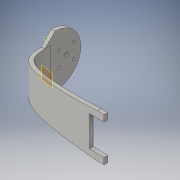
# Autodesk Inventor part: backplaterev2.0
Saved by Autodesk Inventor 2016 (Build 200138000, 138)
## iProperties
Created: 2017-03-21
Part Number: backplaterev2.0
Material: Generic
Document SubType Name: Modeling
Designer: Jorian Bruslind
Density: 1 g/cm^3
Appearance: Default
Author: Jorian Bruslind
Autodesk Inventor part; units mm, degrees
ref_plane "YZ Plane" through (0, 0, 0) normal (1, 0, 0) x (0, 1, 0)
ref_plane "XZ Plane" through (0, 0, 0) normal (0, 1, 0) x (-1, 0, 0)
ref_plane "XY Plane" through (0, 0, 0) normal (0, 0, 1) x (1, 0, 0)
sketch "Sketch5" plane through (0, 0, 0) normal (0, 1, 0) x (-1, 0, 0)
  line L0 (0, 0) -> (82.55, 0) construction
  line L1 (82.55, 0) -> (167.1265, -10.9117) construction
  line L2 (167.1265, -10.9117) -> (165.1, -20.751) construction
  line L3 (165.1, -20.751) -> (165.1, -74.6252) construction
  spline S0 degree 4 poles (0, 0) (82.55, 0) (167.1265, -10.9117) (165.1, -20.751) (165.1, -74.6252) knots 1 1 1 1 1 2 2 2 2 2
  line L4 (165.1, -74.6252) -> (158.7373, -74.6252)
  line L5 (0, 0) -> (0, -6.3627)
  spline S1 degree 5 poles (0, -6.3627) (6.5156, -6.3627) (13.0312, -6.4269) (19.546, -6.5502) (32.2527, -6.903) (44.9512, -7.4802) (51.138, -7.8161) (62.8834, -8.5651) (74.6108, -9.5557) (80.1591, -10.0855) (90.4074, -11.1948) (100.6179, -12.609) (105.2965, -13.3351) (113.6735, -14.8064) (121.9657, -16.6935) (125.6172, -17.6314) (131.9209, -19.4845) (138.0282, -21.9022) (140.5761, -23.0574) (144.8836, -25.3555) (148.7487, -28.32) (150.2858, -29.7215) (153.0054, -32.8262) (154.9786, -36.4507) (155.7539, -38.3472) (157.1958, -42.906) (157.9386, -47.6384) (158.2198, -50.3614) (158.6626, -56.8461) (158.7425, -63.3449) (158.7471, -67.1049) (158.7371, -70.865) (158.7373, -74.6252) knots 0 0 0 0 0 0 0.162165 0.162165 0.162165 0.316364 0.316364 0.316364 0.455071 0.455071 0.455071 0.57289 0.57289 0.57289 0.666676 0.666676 0.666676 0.736221 0.736221 0.736221 0.787638 0.787638 0.787638 0.8383 0.8383 0.8383 0.906414 0.906414 0.906414 1 1 1 1 1 1
  dimension "d24" = 6.3627
  constraints: 4 end point, 1 horizontal, 1 perpendicular, 6 other
extrude "Extrusion4" add sketch "Sketch5" along normal blind 76.2
ref_plane "Work Plane2" through (-105.1206, 76.2, -6.9178) normal (-0.1590682, 0, 0.9872676) x (0, -1, 0)
sketch "Sketch7" plane through (-105.1206, 76.2, -6.9178) normal (-0.1590682, 0, 0.9872676) x (0, -1, 0)
  line L0 (76.2, 104.8825) -> (63.5, 104.8825)
  line L1 (76.2, 104.8825) -> (0, 104.8825) projected
  line L2 (63.5, 104.8825) -> (63.5, -85.6175)
  line L3 (63.5, -85.6175) -> (12.7, -85.6175)
  line L4 (63.5, -85.6175) -> (76.2, 104.8825)
  line L5 (12.7, -85.6175) -> (0, 104.8825)
  line L6 (76.2, 104.8825) -> (0, 104.8825)
  line L7 (0, 104.8825) -> (0, -85.6175)
  line L8 (0, -85.6175) -> (76.2, -85.6175)
  line L9 (76.2, -85.6175) -> (76.2, 104.8825)
  dimension "d27" = 12.7
  dimension "d28" = 190.5
  dimension "d29" = 50.8
  constraints: 18 end point, 2 horizontal, 2 parallel, 2 perpendicular, 1 point on line
  measures "d27" distance of L0.start L0.end
  measures "d28" distance of L0.end L2.end
  measures "d29" distance of L2.end L3.end
extrude "Extrusion5" cut sketch "Sketch7" against normal blind 76.2 contours L9 L8 L4 | L5 L8 L7
ref_plane "Work Plane3" through (-165.1, 64.5421, -74.6252) normal (-1, 0, 0) x (0, -1, 0)
sketch "Sketch8" plane through (-165.1, 64.5421, -74.6252) normal (-1, 0, 0) x (0, -1, 0)
  line L0 (52.8842, 0) -> (0, 0) projected
  line L1 (0, 0) -> (26.4421, 0)
  circle A0 centre (26.4421, 0) radius 44.45
  line L2 (-18.0079, 0) -> (2.3121, 20.32)
  line L3 (50.5721, 20.32) -> (70.8921, 0)
  line L4 (2.3121, 20.32) -> (50.5721, 20.32)
  point P0 (64.5421, 74.6252)
  dimension "d32" = 88.9
  dimension "d90" = 20.32
  constraints: 8 end point, 2 point on circle, 1 centre point, 1 coincident, 1 horizontal, 1 midpoint, 1 perpendicular
  measures "d32" diameter of A0
  measures "d90" distance from line of L4 L1.end
extrude "Extrusion6" add sketch "Sketch8" against normal blind 6.3627 contours A0 L2 L4 L3 picked at (24.8933, -1.1888)
sketch "Sketch10" plane through (0, 0, 0) normal (1, 0, 0) x (0, 0, -1)
  line L0 (0, 0) -> (0, 0.7937)
  line L1 (0, 0) -> (0, 76.2) projected
  line L2 (0, 76.2) -> (0, 75.4126)
  line L3 (0, 75.4126) -> (0, 64.2874)
  line L4 (0, 0.7937) -> (0, 11.9189)
  line L5 (0, 11.9189) -> (7.62, 11.9189)
  line L6 (7.62, 11.9189) -> (7.62, 64.2874)
  line L7 (7.62, 64.2874) -> (0, 64.2874)
  line L8 (0, 64.2874) -> (0, 11.9189)
  line L9 (0, 76.2) -> (7.62, 76.2)
  line L10 (7.62, 76.2) -> (7.62, 75.4126)
  line L11 (7.62, 75.4126) -> (0, 75.4126)
  line L12 (0, 75.4126) -> (0, 76.2)
  line L13 (0, 0.7937) -> (7.62, 0.7937)
  line L14 (7.62, 0.7937) -> (7.62, 0.0064)
  line L15 (7.62, 0.0064) -> (0, 0.0064)
  line L16 (0, 0.0064) -> (0, 0.7937)
  dimension "d47" = 0.7937
  dimension "d48" = 0.7874
  dimension "d49" = 11.1252
  dimension "d50" = 11.1252
  dimension "d51" = 7.62
  dimension "d52" = 7.62
  dimension "d53" = 7.62
  dimension "d54" = 0.7874
  constraints: 32 end point, 6 parallel, 4 point on line, 3 horizontal, 3 perpendicular
  measures "d47" distance of L0.start L0.end
  measures "d48" distance of L1.end L2.end
  measures "d49" distance of L2.end L3.end
  measures "d50" distance of L0.end L4.end
  measures "d51" distance of L7.end L6.end
  measures "d52" distance of L10.end L11.end
  measures "d53" distance of L14.end L15.end
  measures "d54" distance of L13.end L14.end
extrude "Extrusion8" cut sketch "Sketch10" against normal blind 25.4
sketch "Sketch11" plane through (-165.1, 64.5421, -74.6252) normal (-1, 0, 0) x (0, 0, 1)
  arc A0 (0, 18.0079) -> (0, -70.8921) centre (0, -26.4421) ccw projected
  line L0 (0, -70.8921) -> (0, 18.0079)
  line L1 (-165.1, -53.3794) -> (-165.1, 0.4952) projected
  line L2 (0, -26.4421) -> (-19.05, -26.4421)
  line L3 (-19.05, -26.4421) -> (-31.75, -26.4421)
  line L4 (-31.75, -26.4421) -> (-31.75, -13.7421)
  line L5 (-31.75, -26.4421) -> (-31.75, -39.1421)
  circle A1 centre (-31.75, -13.7421) radius 2.5
  circle A2 centre (-31.75, -39.1421) radius 2.5
  circle A3 centre (-19.05, -26.4421) radius 3.81
  line L6 (0, -26.4421) -> (0, -13.7421)
  line L7 (0, -52.8842) -> (0, 0) projected
  line L8 (0, -26.4421) -> (0, -39.1421)
  line L9 (-19.05, -26.4421) -> (-6.35, -26.4421)
  line L10 (-6.35, -39.1421) -> (-6.35, -26.4421)
  line L11 (-6.35, -26.4421) -> (-6.35, -13.7421)
  circle A4 centre (-6.35, -39.1421) radius 2.5
  circle A5 centre (-6.35, -13.7421) radius 2.5
  point P0 (74.6252, -64.5421)
  point P1 (7.2093, -53.3794)
  point P2 (7.2093, 0.4952)
  dimension "d57" = 19.05
  dimension "d58" = 12.7
  dimension "d59" = 12.7
  dimension "d60" = 12.7
  dimension "d65" = 5
  dimension "d66" = 5
  dimension "d69" = 7.62
  dimension "d91" = 12.7
  dimension "d92" = 5
  dimension "d93" = 5
  constraints: 20 end point, 5 centre point, 5 coincident, 5 point on line, 2 perpendicular, 2 vertical, 1 horizontal, 1 vertical alignment
  measures "d57" distance of L2.start L2.end
  measures "d58" distance of L2.end L3.end
  measures "d59" distance of L3.end L4.end
  measures "d60" distance of L3.end L5.end
  measures "d65" diameter of A1
  measures "d66" diameter of A2
  measures "d69" diameter of A3
  measures "d91" distance of L9.start L9.end
  measures "d92" diameter of A4
  measures "d93" diameter of A5
sketch "Sketch12" plane through (-165.1, 64.5421, -74.6252) normal (-1, 0, 0) x (0, -1, 0)
  line L0 (-0.4952, 7.2093) -> (-0.4952, -5.4907)
  circle A0 centre (-0.4952, -5.4907) radius 3.5
  circle A1 centre (-0.4952, -5.4907) radius 4.5
  point P0 (64.5421, 74.6252)
  point P1 (11.6914, 0)
  point P2 (53.3794, 7.2093)
  dimension "d72" = 12.7
  dimension "d73" = 7
  dimension "d74" = 9
  constraints: 2 centre point, 2 coincident, 2 end point, 1 vertical, 1 other
  measures "d72" distance of L0.start L0.end
  measures "d73" diameter of A0
  measures "d74" diameter of A1
extrude "Extrusion11" add sketch "Sketch12" along normal blind 2
sketch "Sketch13" plane through (-167.1, 65.0373, -80.1159) normal (-1, 0, 0) x (0, 0, 1)
  line L0 (0, 0) -> (0, 5.08)
  line L1 (0, 5.08) -> (-0.635, 5.08)
  line L2 (-0.635, 5.08) -> (0.635, 5.08)
  line L3 (0.635, 5.08) -> (0.635, -5.08)
  line L4 (0.635, -5.08) -> (-0.635, -5.08)
  line L5 (-0.635, -5.08) -> (-0.635, 5.08)
  point P0 (80.1159, -65.0373)
  dimension "d82" = 5.08
  dimension "d83" = 0.635
  dimension "d84" = 1.27
  dimension "d85" = 10.16
  constraints: 12 end point, 2 parallel, 2 perpendicular, 1 horizontal, 1 vertical
  measures "d82" distance of L0.start L0.end
  measures "d83" distance of L0.end L1.end
  measures "d84" distance of L3.end L4.end
  measures "d85" distance of L2.end L3.end
extrude "Extrusion12" cut sketch "Sketch13" against normal blind 2
extrude "Extrusion14" cut sketch "Sketch11" against normal blind 6.604 contours A3 L3 L2 | L2 L3 A3 | A1 | A2 | A4 | A5
body "Solid3"
